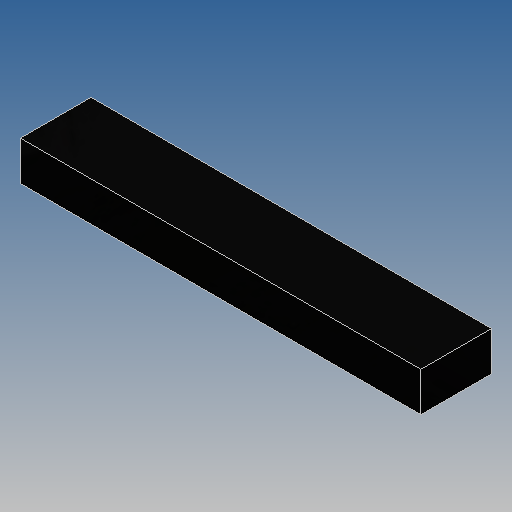
# Autodesk Inventor part: R006
Saved by Autodesk Inventor 2017 (Build 210142000, 142)
## iProperties
Created: 2018-10-19
Part Number: R006
Material: Générique
Document SubType Name: Modeling
Designer: Gilles Mottiez
Density: 1 g/cm^3
Appearance: Anodisé - Noir
Description: GPIO Raspberry pi 3B
Mass: 2.295 g
Surface Area: 15.18 cm^2
Volume: 2.295 cm^3
Author: Gilles Mottiez
Autodesk Inventor part; units mm, degrees
ref_plane "YZ Plane" through (0, 0, 0) normal (1, 0, 0) x (0, 1, 0)
ref_plane "XZ Plane" through (0, 0, 0) normal (0, 1, 0) x (-1, 0, 0)
ref_plane "XY Plane" through (0, 0, 0) normal (0, 0, 1) x (1, 0, 0)
sketch "Sketch1" plane through (0, 0, 0) normal (0, 0, 1) x (1, 0, 0)
  line L0 (0, 0) -> (-51, 0)
  line L1 (-51, 0) -> (-51, -5)
  line L2 (-51, -5) -> (0, -5)
  line L3 (0, -5) -> (0, 0)
  dimension "d0" = 51
  dimension "d1" = 5
  constraints: 8 end point, 2 parallel, 1 horizontal, 1 perpendicular
  measures "d0" distance of L2.end L1.end
  measures "d1" distance of L1.end L0.end
extrude "Extrusion1" add sketch "Sketch1" along normal blind 9
